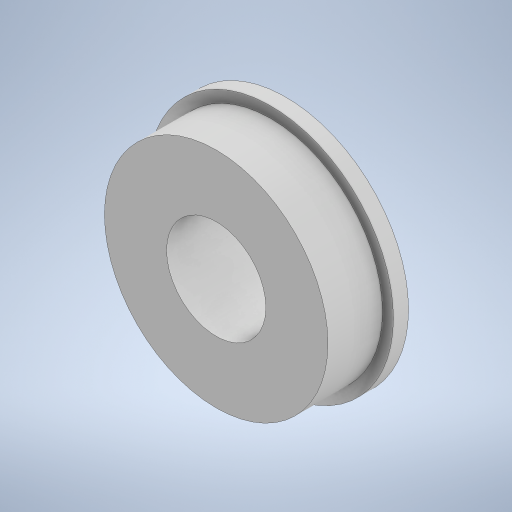
# Autodesk Inventor part: DriveScrewFlangedJournalBearing
Saved by Autodesk Inventor 2024 (Build 280153000, 153)
## iProperties
Created: 2025-01-04
Part Number: DriveScrewFlangedJournalBearing
Material: Generic
Document SubType Name: Modeling
Designer: Tommy Rohmann
Density: 1 g/cm^3
Appearance: Default
Author: Tommy Rohmann
Autodesk Inventor part; units mm, degrees
ref_plane "YZ Plane" through (0, 0, 0) normal (1, 0, 0) x (0, 1, 0)
ref_plane "XZ Plane" through (0, 0, 0) normal (0, 1, 0) x (-1, 0, 0)
ref_plane "XY Plane" through (0, 0, 0) normal (0, 0, 1) x (1, 0, 0)
sketch "Sketch1" plane through (0, 0, 0) normal (0, 0, 1) x (1, 0, 0)
  circle A0 centre (0, 0) radius 14.2875
  circle A1 centre (0, 0) radius 15.6845
  circle A2 centre (0, 0) radius 8.5725
  circle A3 centre (0, 0) radius 6.35
  dimension "d0" = 28.575
  dimension "d1" = 31.369
  dimension "d2" = 17.145
  dimension "d3" = 12.7
  constraints: 4 centre point, 4 coincident
  measures "d0" diameter of A0
  measures "d1" diameter of A1
  measures "d2" diameter of A2
  measures "d3" diameter of A3
extrude "Extrusion1" add sketch "Sketch1" along normal blind 8.9027 contours A0 | A2
extrude "Extrusion2" add sketch "Sketch1" along normal blind 1.9304 contours A1
extrude "Extrusion3" add sketch "Sketch1" against normal blind 1.27 contours A2
body "Solid1"
